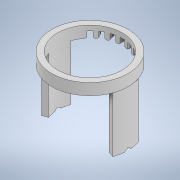
# Autodesk Inventor part: cable_jig_holder
Saved by Autodesk Inventor 2022 (Build 260153000, 153)
## iProperties
Created: 2022-03-09
Part Number: cable_jig_holder
Material: Generic
Document SubType Name: Modeling
Designer: kylem
Density: 1 g/cm^3
Appearance: Default
Author: kylem
Autodesk Inventor part; units mm, degrees
ref_plane "YZ Plane" through (0, 0, 0) normal (1, 0, 0) x (0, 1, 0)
ref_plane "XZ Plane" through (0, 0, 0) normal (0, 1, 0) x (-1, 0, 0)
ref_plane "XY Plane" through (0, 0, 0) normal (0, 0, 1) x (1, 0, 0)
sketch "Sketch1" plane through (0, 0, 0) normal (0, 1, 0) x (-1, 0, 0)
  circle A0 centre (0, 0) radius 35.15
  circle A1 centre (0, 0) radius 29.75
  dimension "d0" = 70.3
  dimension "d1" = 59.5
  constraints: 2 centre point, 2 coincident
  measures "d0" diameter of A0
  measures "d1" diameter of A1
extrude "Extrusion1" add sketch "Sketch1" along normal blind 10.5
sketch "Sketch2" plane through (0, 0, 0) normal (0, -1, 0) x (1, 0, 0)
  line L0 (0, 0) -> (37.5877, -13.6808)
  line L1 (0, 0) -> (40, 0) construction
  line L2 (0, 0) -> (6.8145, 0)
  circle A0 centre (0, 0) radius 29.75
  circle A1 centre (0, 0) radius 34.95
  line L3 (0, 0) -> (37.5877, 13.6808)
  line L4 (0, 0) -> (0, 5.9562)
  line L5 (0, 0) -> (-37.5877, -13.6808)
  line L6 (0, 0) -> (-37.5877, 13.6808)
  point P0 (-32.8423, -11.9536)
  point P1 (-27.9559, -10.1751)
  point P2 (-27.9559, 10.1751)
  point P3 (-32.8423, 11.9536)
  point P4 (32.8423, 11.9536)
  point P5 (27.9559, 10.1751)
  point P6 (27.9559, -10.1751)
  point P7 (32.8423, -11.9536)
  dimension "d4" = 40
  dimension "d5" = 20
  constraints: 14 end point, 3 symmetric about line, 2 centre point, 2 coincident, 1 equal length, 1 horizontal, 1 point on line, 1 vertical
  measures "d4" distance of L0.start L0.end
  measures "d5" angle of L0 L1
extrude "Extrusion2" add sketch "Sketch2" along normal blind 51 contours A0 L3 A1 L0 | L5 A1 L6 A0
sketch "Sketch3" plane through (0, -51, 0) normal (0, -1, 0) x (1, 0, 0)
  arc A0 (-27.9559, 10.1751) -> (-27.9559, -10.1751) centre (0, 0) ccw projected
  circle A1 centre (0, 0) radius 29.75
  arc A2 (-32.8423, 11.9536) -> (-32.8423, -11.9536) centre (0, 0) ccw projected
  circle A3 centre (0, 0) radius 34.95
  line L0 (0, 0) -> (38.637, 10.3528)
  line L1 (0, 0) -> (40, 0) construction
  line L2 (0, 0) -> (-5.4085, 0)
  line L3 (-5.4085, 0) -> (0, 0)
  line L4 (0, 0) -> (0, 7.8245)
  line L5 (0, 0) -> (38.637, -10.3528)
  line L6 (0, 0) -> (-38.637, -10.3528)
  line L7 (0, 0) -> (-33.7591, 9.0457)
  line L8 (-33.7591, 9.0457) -> (-28.7363, 7.6999)
  line L9 (-28.7363, -7.6999) -> (-33.7591, -9.0457)
  circle A4 centre (-31.2477, 8.3728) radius 1.4
  circle A5 centre (-31.2477, -8.3728) radius 1.4
  circle A6 centre (31.2477, 8.3728) radius 1.4
  circle A7 centre (31.2477, -8.3728) radius 1.4
  point P0 (-38.637, 10.3528)
  dimension "d8" = 40
  dimension "d9" = 15
  dimension "d10" = 2.8
  constraints: 20 end point, 6 centre point, 6 point on circle, 6 symmetric about line, 4 point on line, 2 coincident, 1 collinear, 1 equal length, 1 horizontal, 1 midpoint, 1 vertical, 3 other
  measures "d8" distance of L0.start L0.end
  measures "d9" angle of L1 L0
  measures "d10" diameter of A4
extrude "Extrusion3" cut sketch "Sketch3" against normal blind 15 contours A4 L7 | L7 A4 | A6 L0 | L0 A6 | A5 L6 | L6 A5 | A7 L5 | L5 A7
sketch "Sketch4" plane through (0, 0, 0) normal (1, 0, 0) x (0, 1, 0)
  line L0 (-51, 11.9536) -> (-51, -11.9536) projected
  line L1 (-51, 0) -> (-52.5, 0)
  circle A0 centre (-52.5, 0) radius 3.25
  line L2 (-49.25, 0) -> (-48.75, 0)
  line L3 (-48.75, 0) -> (-49.6833, 1.6214)
  line L4 (-48.75, 0) -> (-49.6833, -1.6214)
  point P0 (0, 0)
  point P1 (-51, 2.8831)
  point P2 (-51, -2.8831)
  dimension "d13" = 1.5
  dimension "d14" = 6.5
  dimension "d15" = 0.5
  constraints: 8 end point, 3 point on circle, 2 tangent, 1 centre point, 1 coincident, 1 horizontal, 1 midpoint, 1 perpendicular
  measures "d13" distance of L1.start L1.end
  measures "d14" diameter of A0
  measures "d15" distance of L2.start L2.end
extrude "Extrusion4" cut sketch "Sketch4" along normal mid plane 1500 contours A0 L0 | L3 L2 A0 | L2 L4 A0 picked at (-50.8278, 1.8106)
sketch "Sketch5" plane through (0, 0, 0) normal (0, -1, 0) x (1, 0, 0)
  line L0 (0, 0) -> (2, 0)
  line L1 (2, 0) -> (-2, 0)
  line L2 (-2, 0) -> (-2, -40)
  line L3 (-2, -40) -> (2, -40)
  line L4 (2, -40) -> (2, 0)
  line L5 (0, 0) -> (1.9319, 0.5176)
  line L6 (1.9319, 0.5176) -> (-1.9319, -0.5176)
  line L7 (-1.9319, -0.5176) -> (8.4209, -39.1547)
  line L8 (8.4209, -39.1547) -> (12.2846, -38.1194)
  line L9 (12.2846, -38.1194) -> (1.9319, 0.5176)
  line L10 (0, 0) -> (1.7321, 1)
  line L11 (1.7321, 1) -> (-1.7321, -1)
  line L12 (-1.7321, -1) -> (18.2679, -35.641)
  line L13 (18.2679, -35.641) -> (21.7321, -33.641)
  line L14 (21.7321, -33.641) -> (1.7321, 1)
  line L15 (0, 0) -> (1.4142, 1.4142)
  line L16 (1.4142, 1.4142) -> (-1.4142, -1.4142)
  line L17 (-1.4142, -1.4142) -> (26.8701, -29.6985)
  line L18 (26.8701, -29.6985) -> (29.6985, -26.8701)
  line L19 (29.6985, -26.8701) -> (1.4142, 1.4142)
  line L20 (0, 0) -> (0, 11.8848)
  line L21 (2, 0) -> (2, -40)
  line L22 (2, -40) -> (-2, -40)
  line L23 (-2, -40) -> (-2, 0)
  line L24 (0, 0) -> (-1.9319, 0.5176)
  line L25 (-1.9319, 0.5176) -> (1.9319, -0.5176)
  line L26 (1.9319, -0.5176) -> (-8.4209, -39.1547)
  line L27 (-8.4209, -39.1547) -> (-12.2846, -38.1194)
  line L28 (-12.2846, -38.1194) -> (-1.9319, 0.5176)
  line L29 (0, 0) -> (-1.7321, 1)
  line L30 (-1.7321, 1) -> (1.7321, -1)
  line L31 (1.7321, -1) -> (-18.2679, -35.641)
  line L32 (-18.2679, -35.641) -> (-21.7321, -33.641)
  line L33 (-21.7321, -33.641) -> (-1.7321, 1)
  line L34 (0, 0) -> (-1.4142, 1.4142)
  line L35 (-1.4142, 1.4142) -> (1.4142, -1.4142)
  line L36 (1.4142, -1.4142) -> (-26.8701, -29.6985)
  line L37 (-26.8701, -29.6985) -> (-29.6985, -26.8701)
  line L38 (-29.6985, -26.8701) -> (-1.4142, 1.4142)
  point P0 (9.3278, -12.1562)
  point P1 (-9.3278, -12.1562)
  point P2 (-5.8637, -14.1562)
  point P3 (-2, -15.1915)
  point P4 (2, -15.1915)
  point P5 (5.8637, -14.1562)
  point P6 (3.8637, -6.6921)
  dimension "d18" = 2
  dimension "d19" = 4
  dimension "d20" = 40
  dimension "d23" = 45
  constraints: 78 end point, 16 symmetric about line, 2 horizontal, 2 parallel, 2 perpendicular, 1 coincident, 30 other
  measures "d18" distance of L0.start L0.end
  measures "d19" distance of L3.end L2.end
  measures "d20" distance of L2.end L1.end
extrude "Extrusion5" cut sketch "Sketch5" against normal blind 6 contours L5 L9 L17 L4 L0 | L6 L7 L36 L2 L1 | L11 L12 L36 L7 L6 | L15 L19 L18 L17 L14 L10 | L16 L17 L36 L12 L11 | L35 L36 L17 L16 | L1 L2 L36 L28 L24 | L0 L4 L17 L26 L25 | L24 L28 L36 L33 L29 | L25 L26 L17 L31 L30 | L29 L33 L36 L37 L38 L34 | L30 L31 L17 L36 L35 | L17 L9 L12 L4 | L4 L12 L26 L17 | L36 L7 L31 L2 | L2 L31 L28 L36 | L17 L14 L13 L12 L9 | L36 L12 L31 L7 | L36 L17 L31 L12 | L28 L31 L32 L33 L36 | L26 L12 L31 L17 | L12 L9 L8 L7 L4 | L4 L7 L26 L12 | L31 L7 L26 L2 | L2 L26 L27 L28 L31 | L31 L12 L26 L7 | L4 L3 L2 L26 L7
chamfer "Chamfer1" distance 1 angle 45 14 edges at (24.3159, 0, -21.4875) (21.4875, 0, -24.3159) (17.926, 0, -27.0487) (14.4619, 0, -29.0487) (10.3145, 0, -30.7666) (6.4507, 0, -31.8019) (2, 0, -32.3879) (-2, 0, -32.3879) (-6.4507, 0, -31.8019) (-10.3145, 0, -30.7666) (-14.4619, 0, -29.0487) (-17.926, 0, -27.0487) (-21.4875, 0, -24.3159) (-24.3159, 0, -21.4875)
body "Solid1"
